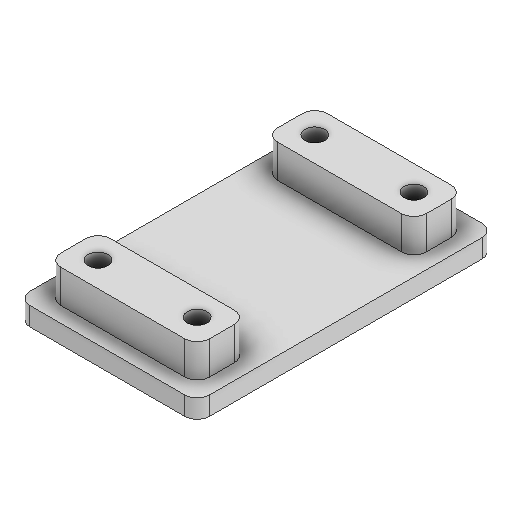
# Autodesk Inventor part: 3DP_ASA_Bias_Tee_Case_Top
Saved by Autodesk Inventor 2026.1 (Build 301233000, 233)
## iProperties
Created: 2025-06-27
Part Number: 3DP_ASA_Bias_Tee_Case_Top
Material: Generic
Document SubType Name: Modeling
Designer: User
Density: 1 g/cm^3
Appearance: Default
Author: User
Autodesk Inventor part; units mm, degrees
ref_plane "YZ Plane" through (0, 0, 0) normal (1, 0, 0) x (0, 1, 0)
ref_plane "XZ Plane" through (0, 0, 0) normal (0, 1, 0) x (-1, 0, 0)
ref_plane "XY Plane" through (0, 0, 0) normal (0, 0, 1) x (1, 0, 0)
sketch "Sketch1" plane through (0, 0, 0) normal (0, 1, 0) x (-1, 0, 0)
  line L0 (12, 21.5) -> (-12, 21.5)
  line L1 (-12, 21.5) -> (-12, -21.5)
  line L2 (-12, -21.5) -> (12, -21.5)
  line L3 (12, -21.5) -> (12, 21.5)
  line L4 (12.5, 22) -> (-12.5, 22)
  line L5 (-12.5, 22) -> (-12.5, -22)
  line L6 (-12.5, -22) -> (12.5, -22)
  line L7 (12.5, -22) -> (12.5, 22)
  line L8 (14.5, 24) -> (-14.5, 24)
  line L9 (-14.5, 24) -> (-14.5, -24)
  line L10 (-14.5, -24) -> (14.5, -24)
  line L11 (14.5, -24) -> (14.5, 24)
  circle A0 centre (8, 17.5) radius 1.6
  circle A1 centre (8, -17.5) radius 1.6
  circle A2 centre (-8, 17.5) radius 1.6
  circle A3 centre (-8, -17.5) radius 1.6
  line L12 (12, -13.5) -> (-12, -13.5)
  line L13 (12, 13.5) -> (-12, 13.5)
  point P0 (0, 0)
  dimension "d0" = 43
  dimension "d1" = 24
  dimension "d2" = 12
  dimension "d3" = 21.5
  dimension "d4" = 4
  dimension "d5" = 4
  dimension "d6" = 4
  dimension "d7" = 4
  dimension "d8" = 0.5
  dimension "d9" = 2
  dimension "d10" = 3.2
  dimension "d11" = 3.2
  dimension "d12" = 3.2
  dimension "d13" = 3.2
  dimension "d45" = 8
  dimension "d46" = 8
  constraints: 28 end point, 7 parallel, 4 centre point, 4 coincident, 4 perpendicular, 4 point on line, 2 horizontal alignment, 2 vertical alignment, 1 horizontal, 6 other
  measures "d0" distance between parallel lines of L2 L0
  measures "d1" distance of L1.end L2.end
  measures "d2" distance from line of L3 point (0, 0)
  measures "d3" distance from line of L2 point (0, 0)
  measures "d4" distance from line of L0 point (8, 17.5)
  measures "d5" distance from line of L3 point (8, 17.5)
  measures "d6" distance from line of L1 point (-8, 17.5)
  measures "d7" distance from line of L2 point (8, -17.5)
  measures "d8" distance between parallel lines of L3 L7
  measures "d9" distance between parallel lines of L7 L11
  measures "d10" diameter of A0
  measures "d11" diameter of A1
  measures "d12" diameter of A2
  measures "d13" diameter of A3
  measures "d45" distance between parallel lines of L2 L12
  measures "d46" distance between parallel lines of L0 L13
extrude "Extrusion1" add sketch "Sketch1" against normal blind 3 contours L3 L13 L1 L0 | L3 L12 L1 L13 | L3 L2 L1 L12 | L7 L6 L5 L4 | L11 L10 L9 L8 | A0 | A1 | A2 | A3
extrude "Extrusion3" cut sketch "Sketch1" against normal blind 6 contours A0 | A1 | A2 | A3
extrude "Extrusion7" add sketch "Sketch1" along normal blind 5.35 contours L3 L13 L1 L0 | L3 L2 L1 L12
fillet "Fillet3" radius 2 4 edges at (14.5, -1.5, 24) (-14.5, -1.5, 24) (14.5, -1.5, -24) (-14.5, -1.5, -24)
fillet "Fillet4" radius 2 8 edges at (12, 2.675, 21.5) (12, 2.675, 13.5) (-12, 2.675, 21.5) (-12, 2.675, 13.5) (12, 2.675, -13.5) (12, 2.675, -21.5) (-12, 2.675, -21.5) (-12, 2.675, -13.5)
equation "\"d2\" = 0.5 * d1"
equation "\"d3\" = 0.5 * d0"
equation "\"d5\" = d4"
equation "\"d6\" = d5"
equation "\"d7\" = d4"
equation "\"d10\" = d13"
equation "\"d11\" = d13"
equation "\"d12\" = d13"
body "Solid1"
